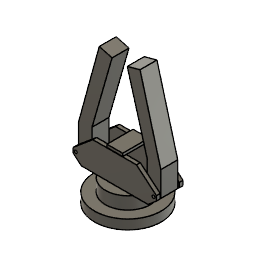
Garra (Autodesk Fusion 360 design; units mm, degrees)
part number: 2026-06-03-19-40-48-217
Autodesk Fusion 360 part; units mm, degrees
sketch "Esboço1" plane through (0, 0, 0) normal (0, 1, 0) x (1, 0, 0)
  line L0 (8.5854, 43.6541) -> (29.1395, -26.3459)
  line L1 (29.1395, -26.3459) -> (38.9697, -24.5105)
  line L2 (38.9697, -24.5105) -> (32.5854, 46.4895)
  line L3 (32.5854, 46.4895) -> (8.5854, 43.6541)
  line L4 (29.1395, -26.3459) -> (24.2245, -27.2636)
  line L5 (24.2245, -27.2636) -> (21.5139, -36.8892)
  line L6 (21.5139, -36.8892) -> (26.3701, -48.9482)
  line L7 (26.3701, -48.9482) -> (30.5265, -78.6588)
  line L8 (30.5265, -78.6588) -> (30.5265, -85.6588)
  line L9 (30.5265, -85.6588) -> (41.5265, -85.6588)
  line L10 (41.5265, -85.6588) -> (41.5265, -35.6588)
  line L11 (41.5265, -35.6588) -> (49.3962, -29.4889)
  line L12 (38.9697, -24.5105) -> (41.7667, -21.7522)
  arc A0 (49.3962, -29.4889) -> (41.7667, -21.7522) centre (47.7431, -23.4889) ccw
  dimension "d1" = 70
  dimension "d2" = 24
  dimension "d3" = 71
  dimension "d10" = 10
  dimension "d11" = 15
  dimension "d12" = 10
  dimension "d13" = 13
  dimension "d14" = 30
  dimension "d15" = 7
  dimension "d16" = 11
  dimension "d17" = 50
  dimension "d18" = 10
  constraint parallel L1 L4
  constraint vertical L8
  constraint perpendicular L8 L9
  constraint perpendicular L9 L10
  measures "d1" vertical distance of L0.start L0.end
  measures "d2" horizontal distance of L0.start L2.end
  measures "d3" vertical distance of L1.end L2.end
  measures "d10" distance of L0.end L1.end
  measures "d11" distance of L1.end L4.end
  measures "d12" distance of L4.end L5.end
  measures "d13" distance of L5.end L6.end
  measures "d14" distance of L6.end L7.end
  measures "d15" distance of L7.end L8.end
  measures "d16" distance of L8.end L9.end
  measures "d17" distance of L9.end L10.end
  measures "d18" distance of L10.end L11.end
sketch "Esboço2" plane through (0, 12.5, 0) normal (0, 1, 0) x (-1, 0, 0)
  line L0 (-38.9697, 24.5105) -> (-32.5854, -46.4895)
  line L1 (-32.5854, -46.4895) -> (-8.5854, -43.6541)
  line L2 (-8.5854, -43.6541) -> (-29.1395, 26.3459)
  line L3 (-29.1395, 26.3459) -> (-24.2245, 27.2636)
  line L4 (-24.2245, 27.2636) -> (-21.5139, 36.8892)
  line L5 (-21.5139, 36.8892) -> (-26.3701, 48.9482)
  line L6 (-26.3701, 48.9482) -> (-30.5265, 78.6588)
  line L7 (-30.5265, 78.6588) -> (-30.5265, 85.6588)
  line L8 (-30.5265, 85.6588) -> (-41.5265, 85.6588)
  line L9 (-41.5265, 85.6588) -> (-41.5265, 35.6588)
  line L10 (-41.5265, 35.6588) -> (-49.3962, 29.4889)
  arc A0 (-49.3962, 29.4889) -> (-41.7667, 21.7522) centre (-47.7431, 23.4889) ccw
  line L11 (-41.7667, 21.7522) -> (-38.9697, 24.5105)
  line L12 (-38.1267, 80.1359) -> (-38.1267, 55.3747)
  line L13 (-38.1267, 55.3747) -> (-28.0919, 55.3747)
  line L14 (-28.0919, 55.3747) -> (-38.1267, 80.1359)
  constraint perpendicular L9 L13
ref_plane "Plano de trabalho1" through (31.1795, -9.5761, 22.915) normal (0.678463, -0.707107, -0.199217) x (-0.730355, -0.678463, -0.079176)
mirror "Espelhar1" [no effect]
sketch "Esboço3" plane through (0, 0, 0) normal (0, 1, 0) x (1, 0, 0)
  circle A0 centre (0, 0) radius 35
  dimension "d40" = 70
  constraint coincident A0.centre origin
  measures "d40" diameter of A0
extrude "Extrusão4" add sketch "Esboço3" along normal blind 10 makes body 1
sketch "Esboço5" plane through (0, 10, 0) normal (0, 1, 0) x (-1, 0, 0)
  circle A0 centre (0, 0) radius 35
  circle A1 centre (0, 0) radius 23.5
  constraint coincident A0.centre A1.centre
extrude "Extrusão5" add sketch "Esboço5" along normal blind 13 contours A1 bodies 1
sketch "Esboço6" plane through (0, 0, 0) normal (0, 0, 1) x (1, 0, 0)
  line L0 (0.1552, 23.1183) -> (35.1552, 23.1183)
  line L1 (35.1552, 23.1183) -> (45.1552, 23.1183)
  line L2 (35.1552, 23.1183) -> (43.9647, 30.5103)
  line L3 (43.9647, 30.5103) -> (43.9647, 35.5103)
  line L4 (0.1552, 23.1183) -> (0.1552, 60.1183)
  line L5 (23.1183, 23.1183) -> (23.1183, 63.1183)
  line L6 (43.9647, 35.5103) -> (23.1183, 53.0025)
  line L7 (43.9647, 35.5103) -> (43.9647, 47.0021)
  line L8 (23.1183, 53.0025) -> (0.1552, 53.0025)
  line L9 (0.1552, 23.1183) -> (-34.8448, 23.1183)
  line L10 (-34.8448, 23.1183) -> (-43.6544, 30.5103)
  line L11 (-43.6544, 30.5103) -> (-43.6544, 35.5103)
  line L12 (-43.6544, 35.5103) -> (-22.808, 53.0025)
  line L13 (-22.808, 53.0025) -> (0.1552, 53.0025)
  dimension "d46" = 35
  dimension "d47" = 10
  dimension "d48" = 11.5
  dimension "d49" = 40
  dimension "d50" = 5
  dimension "d51" = 37
  dimension "d52" = 40
  dimension "d53" = 50
  constraint horizontal L0
  constraint parallel L0 L1
  constraint vertical L3
  constraint perpendicular L0 L4
  constraint coincident L0 L5.start
  constraint perpendicular L0 L5
  constraint coincident L5 L6.end
  constraint parallel L3 L7
  constraint coincident L4 L8.end
  constraint perpendicular L4 L8
  constraint symmetric L0.start L4 L9.start
  constraint symmetric L0.end L4 L9.end
  constraint symmetric L2.end L4 L10.end
  constraint symmetric L3.end L4 L11.end
  constraint symmetric L4 L6.end L12.end
  constraint symmetric L4 L8.end L13.end
  measures "d46" distance of L0.start L0.end
  measures "d47" distance of L0.end L1.end
  measures "d48" distance of L0.end L2.end
  measures "d49" angle of L1 L2
  measures "d50" distance of L2.end L3.end
  measures "d51" distance of L0.start L4.end
  measures "d52" distance of L5.start L5.end
  measures "d53" angle of L6 L7
extrude "Extrusão6" add sketch "Esboço6" against normal blind 4 separate body makes body 2
sketch "Esboço7" plane through (0, 0, 0) normal (0, 0, 1) x (1, 0, 0)
  line L0 (-34.8448, 23.1183) -> (35.1552, 23.1183)
  line L1 (35.1552, 23.1183) -> (43.9647, 30.5103)
  line L2 (43.9647, 30.5103) -> (43.9647, 35.5103)
  line L3 (43.9647, 35.5103) -> (23.1183, 53.0025)
  line L4 (23.1183, 53.0025) -> (-22.808, 53.0025)
  line L5 (-22.808, 53.0025) -> (-43.6544, 35.5103)
  line L6 (-43.6544, 35.5103) -> (-43.6544, 30.5103)
  line L7 (-43.6544, 30.5103) -> (-34.8448, 23.1183)
  line L8 (-43.6544, 33.0103) -> (-40.6544, 33.0103)
  circle A0 centre (-40.6544, 33.0103) radius 1.5
  dimension "d56" = 3
  dimension "d58" = 3
  constraint midpoint L6 L8.start
  constraint perpendicular L6 L8
  constraint coincident L8.end A0.centre
  measures "d56" distance of L8.start L8.end
  measures "d58" diameter of A0
extrude "Extrusão7" cut sketch "Esboço7" against normal blind 8 contours A0 bodies 2
sketch "Esboço8" plane through (0, 0, 0) normal (0, 0, 1) x (1, 0, 0)
  circle A0 centre (-40.6544, 33.0103) radius 1.5
  line L0 (-34.8448, 23.1183) -> (35.1552, 23.1183)
  line L1 (35.1552, 23.1183) -> (43.9647, 30.5103)
  line L2 (43.9647, 30.5103) -> (43.9647, 35.5103)
  line L3 (43.9647, 35.5103) -> (23.1183, 53.0025)
  line L4 (23.1183, 53.0025) -> (-22.808, 53.0025)
  line L5 (-22.808, 53.0025) -> (-43.6544, 35.5103)
  line L6 (-43.6544, 35.5103) -> (-43.6544, 30.5103)
  line L7 (-43.6544, 30.5103) -> (-34.8448, 23.1183)
  line L8 (43.9647, 33.0103) -> (40.9647, 33.0103)
  circle A1 centre (40.9647, 33.0103) radius 1.5
  dimension "d61" = 3
  dimension "d62" = 3
  constraint midpoint L2 L8.start
  constraint perpendicular L2 L8
  constraint coincident L8.end A1.centre
  measures "d61" distance of L8.start L8.end
  measures "d62" diameter of A1
extrude "Extrusão8" cut sketch "Esboço8" against normal blind 11 contours A1 bodies 2
mirror "Espelhar2" about plane through (0, 0, 0) normal (0, 0, 1) of "Extrusão6", "Extrusão7", "Extrusão8" makes body 3
move_body "Mover23" bodies 3 to x (1, 0, 0) y (0, 1, 0) z (0, 0, 1) at (0, -15, 0)
move_body "Mover24" bodies 3 to x (1, 0, 0) y (0, 1, 0) z (0, 0, 1) at (0, 0, 10)
move_body "Mover25" bodies 2 to x (1, 0, 0) y (0, 1, 0) z (0, 0, 1) at (0, 0, -10)
move_body "Mover26" bodies 3 to x (1, 0, 0) y (0, 1, 0) z (0, 0, 1) at (0, 15, 0)
sketch "Esboço11" plane through (0, 53.0025, 0) normal (0, 1, 0) x (-1, 0, 0)
  line L0 (-23.1183, 10) -> (22.808, 10)
  line L1 (22.808, 10) -> (22.808, 14)
  line L2 (22.808, 14) -> (-23.1183, 14)
  line L3 (-23.1183, 14) -> (-23.1183, 10)
  line L4 (8.2465, -13.6976) -> (-8.2465, -13.6976)
  line L5 (-8.2465, -13.6976) -> (-8.2465, 13.6976)
  line L6 (-8.2465, 13.6976) -> (8.2465, 13.6976)
  line L7 (8.2465, 13.6976) -> (8.2465, -13.6976)
  line L8 (8.2465, -13.6976) -> (-8.2465, 13.6976) construction
  line L9 (-8.2465, -13.6976) -> (8.2465, 13.6976) construction
  constraint horizontal L4
  constraint perpendicular L4 L5
  constraint parallel L4 L6
  constraint parallel L5 L7
  constraint coincident L8 origin
  constraint coincident L9 origin
extrude "Extrusão9" add sketch "Esboço11" along normal blind 3 contours L0 L5 L6 L7 | L0 L4 L5 L7 bodies 2 3
sketch "Esboço12" plane through (0, 0, 14) normal (0, 0, 1) x (1, 0, 0)
  circle A0 centre (-40.6544, 33.0103) radius 1.5
  line L0 (-34.8448, 23.1183) -> (35.1552, 23.1183)
  line L1 (35.1552, 23.1183) -> (43.9647, 30.5103)
  line L2 (23.1183, 53.0025) -> (-22.808, 53.0025)
  line L3 (-22.808, 53.0025) -> (-43.6544, 35.5103)
  line L4 (-43.6544, 35.5103) -> (-43.6544, 30.5103)
  line L5 (-43.6544, 30.5103) -> (-34.8448, 23.1183)
  line L6 (35.1552, 23.1183) -> (35.1552, 50.7537)
  line L7 (35.1552, 50.7537) -> (16.794, 117.9533)
  line L8 (16.794, 117.9533) -> (5.4402, 114.851)
  line L9 (5.4402, 114.851) -> (23.1183, 53.0025)
  line L10 (23.1183, 23.1183) -> (35.1552, 23.1183)
  line L11 (23.1183, 23.1183) -> (23.1183, 53.0025)
  constraint coincident L0.end L1.start
  constraint perpendicular L0 L6
  constraint perpendicular L7 L8
  constraint coincident L2.start L9.end
  constraint coincident L0 L10.start
  constraint perpendicular L2 L11
sketch "Esboço14" plane through (0, 56.0025, 0) normal (0, 1, 0) x (-1, 0, 0)
  line L0 (8.2465, 13.6976) -> (-8.2465, 13.6976)
  line L1 (-8.2465, 13.6976) -> (-8.2465, -13.6976)
  line L2 (-8.2465, -13.6976) -> (8.2465, -13.6976)
  line L3 (8.2465, -13.6976) -> (8.2465, 13.6976)
extrude "Extrusão11" add sketch "Esboço12" along normal blind 15 separate body contours L0 L6 L7 L8 L9 L10 L11 makes body 4
move_body "Mover68" bodies 4 to x (1, 0, 0) y (0, 1, 0) z (0, 0, 1) at (0, 0, -18)
move_body "Mover69" bodies 4 to x (1, 0, 0) y (0, 1, 0) z (0, 0, 1) at (0, 0, -5)
scale "Escala3" factor 1.2 about (23.1183, 53.0025, -9) bodies 4
scale "Escala4" factor 1.1 about (23.1183, 53.0025, -9) bodies 4
move_body "Mover70" bodies 4 to x (1, 0, 0) y (0, 1, 0) z (0, 0, 1) at (0, 0, -1)
move_body "Mover71" bodies 4 to x (1, 0, 0) y (0, 1, 0) z (0, 0, 1) at (0, 10, 0)
move_face "MoverFace2" by (-10, 0, 0) 1 faces at (12.5573, 118.7942, -10) on bodies 4
move_body "Mover72" bodies 4 to x (1, 0, 0) y (0, 1, 0) z (0, 0, 1) at (-5, 0, 0)
copy_body "Copiar e colar corpos4" bodies 4 makes body 5
move_body "Mover73" bodies 5 to x (1, 0, 0) y (0, 1, 0) z (0, 0, 1) at (0, 0, 0)
move_body "Mover74" bodies 5 to x (-1, 0, 0) y (0, 1, 0) z (0, 0, -1) at (4.5665, 0, -20)
move_body "Mover75" bodies 5 to x (1, 0, 0) y (0, 1, 0) z (0, 0, 1) at (-5, 0, 20)
scale "Escala5" factor 0.9 about (18.1183, 63.0025, -10) bodies 4
scale "Escala6" factor 0.9 about (-18.5518, 63.0025, -9.8) bodies 5
move_body "Mover76" bodies 4 to x (1, 0, 0) y (0, 1, 0) z (0, 0, 1) at (10, 0, 1)
move_body "Mover77" bodies 5 to x (1, 0, 0) y (0, 1, 0) z (0, 0, 1) at (-10, 0, 1)
move_body "Mover78" bodies 4 to x (1, 0, 0) y (0, 1, 0) z (0, 0, 1) at (3, 0, 0)
move_body "Mover79" bodies 4 to x (1, 0, 0) y (0, 1, 0) z (0, 0, 1) at (-5, 0, 0)
move_body "Mover80" bodies 5 to x (1, 0, 0) y (0, 1, 0) z (0, 0, 1) at (5, 0, 0)
move_body "Mover81" bodies 4 to x (1, 0, 0) y (0, 1, 0) z (0, 0, 1) at (-2, 0, 0)
move_body "Mover82" bodies 4 5 to x (1, 0, 0) y (0, 1, 0) z (0, 0, 1) at (0, -4, 0)
move_body "Mover83" bodies 4 to x (1, 0, 0) y (0, 1, 0) z (0, 0, 1) at (5, 0, 0)
move_body "Mover84" bodies 5 to x (1, 0, 0) y (0, 1, 0) z (0, 0, 1) at (-5, 0, 0)
sketch "Esboço16" plane through (0, 0, 8.82) normal (0, 0, 1) x (1, 0, 0)
  line L0 (43.4181, 23.5) -> (43.4181, 56.331)
  line L1 (43.4181, 56.331) -> (21.6051, 136.164)
  line L2 (21.6051, 136.164) -> (8.1167, 132.4785)
  line L3 (8.1167, 132.4785) -> (29.1183, 59.0025)
  line L4 (29.1183, 59.0025) -> (29.1183, 23.5)
  line L5 (29.1183, 23.5) -> (43.4181, 23.5)
  line L6 (43.4181, 23.5) -> (43.4181, 30.1195)
  line L7 (35.521, 23.5) -> (43.4181, 23.5)
  line L8 (35.521, 23.5) -> (43.4181, 30.1195)
  constraint coincident L0.start L5.end
  constraint coincident L0 L6.end
  constraint coincident L5 L7.start
extrude "Extrusão12" cut sketch "Esboço16" against normal blind 18 contours L0 L5 L6 L7 L8 bodies 4
sketch "Esboço17" plane through (0, 0, 9.02) normal (0, 0, 1) x (1, 0, 0)
  line L0 (-42.8516, 56.331) -> (-42.8516, 23.5)
  line L1 (-42.8516, 23.5) -> (-28.5518, 23.5)
  line L2 (-28.5518, 23.5) -> (-28.5518, 59.0025)
  line L3 (-28.5518, 59.0025) -> (-7.5503, 132.4785)
  line L4 (-7.5503, 132.4785) -> (-21.0386, 136.164)
  line L5 (-21.0386, 136.164) -> (-42.8516, 56.331)
  line L6 (-35.3221, 23.5) -> (-42.8516, 23.5)
  line L7 (-42.8516, 29.578) -> (-35.3221, 23.5)
  constraint coincident L1 L6.start
  constraint coincident L0.end L1.start
  constraint coincident L0 L7.start
extrude "Extrusão13" cut sketch "Esboço17" against normal blind 18 contours L0 L1 L6 L7 bodies 5
sketch "Esboço19" plane through (0, 0, -8.8) normal (0, 0, -1) x (-1, 0, 0)
  line L0 (35.3221, 23.5) -> (42.8516, 29.578)
  line L1 (42.8516, 29.578) -> (42.8516, 56.331)
  line L2 (42.8516, 56.331) -> (21.0386, 136.164)
  line L3 (21.0386, 136.164) -> (7.5503, 132.4785)
  line L4 (7.5503, 132.4785) -> (28.5518, 59.0025)
  line L5 (28.5518, 59.0025) -> (28.5518, 23.5)
  line L6 (28.5518, 23.5) -> (35.3221, 23.5)
  circle A0 centre (40.6062, 32.9312) radius 1.5
  dimension "d92" = 3
  measures "d92" diameter of A0
extrude "Extrusão14" cut sketch "Esboço19" against normal blind 18 contours A0 bodies 5
sketch "Esboço20" plane through (0, 0, -9) normal (0, 0, -1) x (-1, 0, 0)
  line L0 (-43.4181, 30.1195) -> (-35.521, 23.5)
  line L1 (-35.521, 23.5) -> (-29.1183, 23.5)
  line L2 (-29.1183, 23.5) -> (-29.1183, 59.0025)
  line L3 (-29.1183, 59.0025) -> (-8.1167, 132.4785)
  line L4 (-8.1167, 132.4785) -> (-21.6051, 136.164)
  line L5 (-21.6051, 136.164) -> (-43.4181, 56.331)
  line L6 (-43.4181, 56.331) -> (-43.4181, 30.1195)
  circle A0 centre (-40.8071, 33.061) radius 1.5
  dimension "d95" = 3
  measures "d95" diameter of A0
extrude "Extrusão15" cut sketch "Esboço20" against normal blind 19 contours A0 bodies 4
named bodies: "Base", "Suporte", "Garra1", "Garra2"
